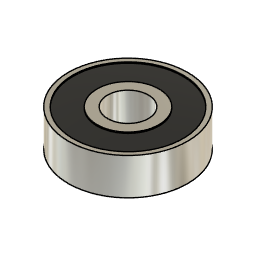
bearing (Autodesk Fusion 360 design; units mm, degrees)
Autodesk Fusion 360 part; units mm, degrees
sketch "main" plane through (0, 0, 0) normal (0, 0, 1) x (1, 0, 0) in component "bearing"
  circle A0 centre (0, 0) radius 13
  circle A1 centre (0, 0) radius 12
  circle A2 centre (0, 0) radius 4.45
  circle A3 centre (0, 0) radius 6.75
  dimension "d1" = 26
  dimension "d2" = 24
  dimension "d3" = 8.9
  dimension "d4" = 13.5
  constraint coincident A0.centre A1.centre
  constraint concentric A0 A1
  constraint concentric A1 A2
  measures "d1" diameter of A0
  measures "d2" diameter of A1
  measures "d3" diameter of A2
  measures "d4" diameter of A3
extrude "Extrude1" add sketch "main" along normal blind 8 makes body 1 at (12.9838, -0.648, 5.3333) makes body 2 at (6.7416, -0.3365, 5.3333) in component "bearing"
extrude "Extrude2" add sketch "main" along normal blind 7.5 from surface at 0.25 separate body contours A1 makes body 3 in component "bearing"
component "bearing" placed x (1, 0, 0) y (0, 1, 0) z (0, 0, 1) at (0, 0, 0)
equation "d2 = 26 mm - 2 mm"
equation "d8 = 8 mm - 0.5 mm"
named bodies: "outer-metal", "inner-metal", "ball-holder"
